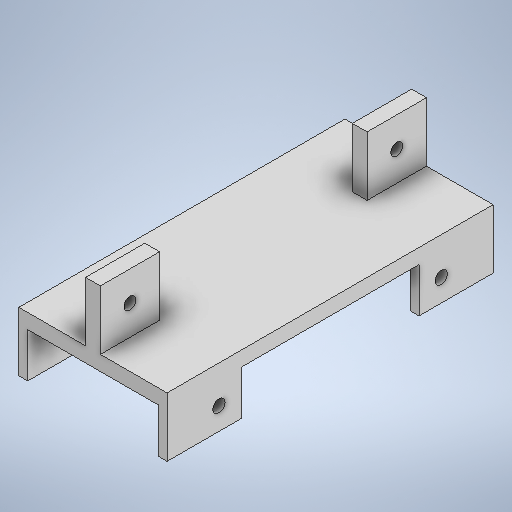
# Autodesk Inventor part: gripper_case_bracket
Saved by Autodesk Inventor 2026.1 (Build 301233000, 233)
## iProperties
Created: 2026-05-21
Part Number: gripper_case_bracket
Material: Generic
Document SubType Name: Modeling
Designer: chris
Density: 1 g/cm^3
Appearance: Default
Author: chris
Autodesk Inventor part; units mm, degrees
ref_plane "YZ Plane" through (0, 0, 0) normal (1, 0, 0) x (0, 1, 0)
ref_plane "XZ Plane" through (0, 0, 0) normal (0, 1, 0) x (-1, 0, 0)
ref_plane "XY Plane" through (0, 0, 0) normal (0, 0, 1) x (1, 0, 0)
sketch "Sketch1" plane through (0, 0, 0) normal (0, 1, 0) x (-1, 0, 0)
  line L0 (25, 55) -> (-25, 55)
  line L1 (-25, 55) -> (-25, -55)
  line L2 (-25, -55) -> (25, -55)
  line L3 (25, -55) -> (25, 55)
  line L4 (25, 55) -> (-25, -55) construction
  line L5 (-25, 55) -> (25, -55) construction
  point P0 (0, 0)
  dimension "d0" = 50
  dimension "d1" = 110
  constraints: 12 end point, 2 midpoint, 2 parallel, 1 horizontal, 1 perpendicular
  measures "d0" distance of L2.end L1.end
  measures "d1" distance of L0.end L1.end
extrude "Extrusion1" add sketch "Sketch1" along normal blind 5
sketch "Sketch2" plane through (0, 0, 0) normal (0, -1, 0) x (1, 0, 0)
  line L0 (25, 55) -> (25, -55) projected
  line L1 (-25, 55) -> (25, 55) projected
  line L2 (-25, -55) -> (-25, 55) projected
  line L3 (25, -55) -> (-25, -55) projected
  line L4 (25, 55) -> (22, 55)
  line L5 (22, 55) -> (22, 30)
  line L6 (22, 30) -> (25, 30)
  line L7 (25, 30) -> (25, 55)
  line L8 (-25, 55) -> (-22, 55)
  line L9 (-22, 55) -> (-22, 30)
  line L10 (-22, 30) -> (-25, 30)
  line L11 (-25, 30) -> (-25, 55)
  line L12 (25, -55) -> (22, -55)
  line L13 (22, -55) -> (22, -30)
  line L14 (22, -30) -> (25, -30)
  line L15 (25, -30) -> (25, -55)
  line L16 (-25, -55) -> (-22, -55)
  line L17 (-22, -55) -> (-22, -30)
  line L18 (-22, -30) -> (-25, -30)
  line L19 (-25, -30) -> (-25, -55)
  point P0 (0, 0)
  dimension "d4" = 3
  dimension "d5" = 3
  dimension "d6" = 3
  dimension "d7" = 25
  dimension "d8" = 25
  dimension "d9" = 25
  dimension "d10" = 25
  constraints: 32 end point, 8 parallel, 4 horizontal, 4 perpendicular, 1 point on line
  measures "d4" distance of L5.end L6.end
  measures "d5" distance of L9.end L10.end
  measures "d6" distance of L17.end L18.end
  measures "d7" distance of L4.end L5.end
  measures "d8" distance of L8.end L9.end
  measures "d9" distance of L16.end L17.end
  measures "d10" distance of L12.end L13.end
extrude "Extrusion2" add sketch "Sketch2" along normal blind 15 contours L0 L6 L5 L1 | L0 L3 L13 L14 | L9 L10 L2 L1 | L3 L2 L18 L17
sketch "Sketch3" plane through (25, 5, 55) normal (1, 0, 0) x (0, 0, -1)
  circle A0 centre (17.5, -12.5) radius 2.05
  circle A1 centre (92.5, -12.5) radius 2.05
  line L0 (25, -20) -> (0, -20) projected
  line L1 (110, -20) -> (85, -20) projected
  line L2 (85, -5) -> (85, -20) projected
  line L3 (25, -5) -> (25, -20) projected
  point P0 (55, -5)
  dimension "d13" = 4.1
  dimension "d14" = 4.1
  dimension "d15" = 7.5
  dimension "d16" = 7.5
  dimension "d17" = 7.5
  dimension "d18" = 7.5
  constraints: 2 centre point
  measures "d13" diameter of A0
  measures "d14" diameter of A1
  measures "d15" distance from line of L0 A0.centre
  measures "d16" distance from line of L1 A1.centre
  measures "d17" distance from line of L2 A1.centre
  measures "d18" distance from line of L3 A0.centre
extrude "Extrusion3" cut sketch "Sketch3" against normal through all
sketch "Sketch5" plane through (0, 0, 0) normal (1, 0, 0) x (0, 1, 0)
  line L0 (25, 55) -> (5, 55)
  line L1 (5, 55) -> (5, 35)
  line L2 (5, 35) -> (25, 35)
  line L3 (25, 35) -> (25, 55)
  line L4 (25, -35) -> (5, -35)
  line L5 (5, -35) -> (5, -55)
  line L6 (5, -55) -> (25, -55)
  line L7 (25, -55) -> (25, -35)
  line L8 (5, 55) -> (5, -55) projected
  line L9 (-15, -55) -> (5, -55) projected
  line L10 (5, 55) -> (-15, 55) projected
  point P0 (0, 0)
  dimension "d21" = 20
  dimension "d22" = 20
  dimension "d23" = 20
  dimension "d24" = 20
  constraints: 16 end point, 4 collinear, 4 parallel, 2 horizontal, 2 perpendicular
  measures "d21" distance of L2.end L0.start
  measures "d22" distance of L1.end L2.end
  measures "d23" distance of L4.start L4.end
  measures "d24" distance of L6.end L4.start
extrude "Extrusion4" add sketch "Sketch5" along normal mid plane 5
sketch "Sketch6" plane through (2.5, 0, 0) normal (1, 0, 0) x (0, 0, -1)
  line L0 (-35, 5) -> (-55, 5) projected
  line L1 (-35, 5) -> (-35, 25) projected
  line L2 (-35, 25) -> (-55, 25) projected
  line L3 (-55, 25) -> (-55, 5) projected
  line L4 (35, 25) -> (35, 5) projected
  line L5 (55, 5) -> (35, 5) projected
  line L6 (55, 5) -> (55, 25) projected
  line L7 (55, 25) -> (35, 25) projected
  circle A0 centre (-45, 15) radius 2
  circle A1 centre (45, 15) radius 2
  point P0 (0, 0)
  dimension "d29" = 4
  dimension "d30" = 4
  constraints: 2 centre point
  measures "d29" diameter of A0
  measures "d30" diameter of A1
extrude "Extrusion5" cut sketch "Sketch6" against normal blind 5 contours A0 | A1
body "Solid1"
